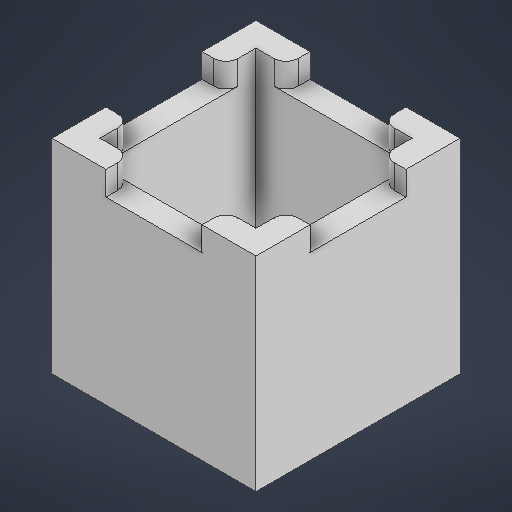
# Autodesk Inventor part: reference_magnet_box
Saved by Autodesk Inventor 2026.1 (Build 301233020, 233B)
## iProperties
Created: 2025-11-29
Part Number: reference_magnet_box
Material: Generic
Document SubType Name: Modeling
Designer: Carla Fernandez
Density: 1 g/cm^3
Appearance: Default
Author: Carla Fernandez
Autodesk Inventor part; units mm, degrees
ref_plane "YZ Plane" through (0, 0, 0) normal (1, 0, 0) x (0, 1, 0)
ref_plane "XZ Plane" through (0, 0, 0) normal (0, 1, 0) x (-1, 0, 0)
ref_plane "XY Plane" through (0, 0, 0) normal (0, 0, 1) x (1, 0, 0)
sketch "Sketch1" plane through (0, 0, 0) normal (0, 1, 0) x (-1, 0, 0)
  line L0 (8.5, 8.5) -> (-8.5, 8.5)
  line L1 (-8.5, 8.5) -> (-8.5, -8.5)
  line L2 (-8.5, -8.5) -> (8.5, -8.5)
  line L3 (8.5, -8.5) -> (8.5, 8.5)
  line L4 (6.5, 6.5) -> (-6.5, 6.5) construction
  line L5 (-6.5, 6.5) -> (-6.5, -6.5) construction
  line L6 (-6.5, -6.5) -> (6.5, -6.5) construction
  line L7 (6.5, -6.5) -> (6.5, 6.5) construction
  point P0 (0, 0)
  point P1 (8.5, 0)
  point P2 (0, -6.5)
  point P3 (0, -8.5)
  point P4 (6.5, 0)
  dimension "d0" = 13
  dimension "d1" = 13
  dimension "d2" = 17
  constraints: 16 end point, 4 midpoint, 4 parallel, 3 perpendicular, 2 horizontal, 2 horizontal alignment, 2 vertical alignment
  measures "d0" distance of L6.end L4.start
  measures "d1" distance of L5.end L6.end
  measures "d2" distance of L0.start L0.end
extrude "Extrusion1" add sketch "Sketch1" along normal blind 17
shell "Shell1" thickness 2 removed faces 1 at (2.8333, 17, 2.8333)
sketch "Sketch2" plane through (0, 17, 0) normal (0, 1, 0) x (1, 0, 0)
  line L0 (6, -4) -> (8.5, -4)
  line L1 (4, -6) -> (4, -8.5)
  line L2 (0, -12.5225) -> (0, 10.2466) construction
  line L3 (-9.8637, 0) -> (11.1563, 0) construction
  line L4 (4, -8.5) -> (0, -8.5)
  line L5 (0, -8.5) -> (4, -8.5) construction
  line L6 (-8.5, -8.5) -> (8.5, -8.5) construction
  line L7 (6, 4) -> (8.5, 4)
  line L8 (8.5, 4) -> (8.5, 0)
  line L9 (4, 6) -> (4, 8.5)
  line L10 (4, 8.5) -> (0, 8.5)
  line L11 (8.5, -4) -> (8.5, 4)
  line L12 (-6, -4) -> (-8.5, -4)
  line L13 (-4, -6) -> (-4, -8.5)
  line L14 (-4, -8.5) -> (0, -8.5)
  line L15 (-4, 8.5) -> (0, 8.5)
  line L16 (-4, 6) -> (-4, 8.5)
  line L17 (-6, 4) -> (-8.5, 4)
  line L18 (-8.5, 4) -> (-8.5, 0)
  line L19 (-8.5, -4) -> (-8.5, 4)
  arc A0 (-4, -6) -> (-6, -4) centre (-6, -6) ccw
  arc A1 (-6, 4) -> (-4, 6) centre (-6, 6) ccw
  arc A2 (4, 6) -> (6, 4) centre (6, 6) ccw
  arc A3 (6, -4) -> (4, -6) centre (6, -6) ccw
  point P0 (0, 0)
  point P1 (4, -4)
  point P2 (4, 4)
  point P3 (-4, -4)
  point P4 (-11.1563, 0)
  point P5 (-4, 4)
  dimension "d6" = 4
  dimension "d7" = 4
  dimension "d8" = 2
  constraints: 38 end point, 12 symmetric about line, 11 point on line, 8 point on circle, 8 tangent, 4 centre point, 3 equal radius, 2 horizontal, 1 collinear, 1 vertical
  measures "d6" distance between parallel lines of L0 L3
  measures "d7" distance between parallel lines of L1 L2
  measures "d8" radius of A0
extrude "Extrusion2" cut sketch "Sketch2" against normal blind 2
fillet "Fillet1" radius 1 8 edges at (-6.5, 16, 4) (-4, 16, 6.5) (-6.5, 16, -4) (-4, 16, -6.5) (4, 16, -6.5) (6.5, 16, -4) (6.5, 16, 4) (4, 16, 6.5)
equation "\"d3\" = d2"
equation "\"d7\" = d6"
body "Solid1"
